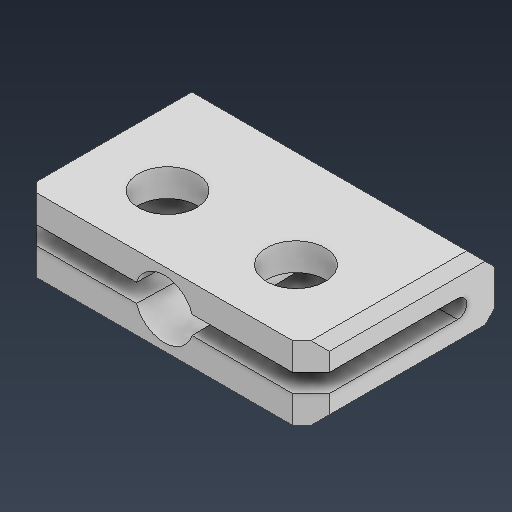
# Autodesk Inventor part: Sup_haste_corpo
Saved by Autodesk Inventor 2026.1 (Build 301233020, 233B)
## iProperties
Created: 2026-03-23
Part Number: Sup_haste_corpo
Material: Genérico
Document SubType Name: Modeling
Designer: celio
Density: 1 g/cm^3
Appearance: Padrão
Author: celio
Autodesk Inventor part; units mm, degrees
ref_plane "YZ Plane" through (0, 0, 0) normal (1, 0, 0) x (0, 1, 0)
ref_plane "XZ Plane" through (0, 0, 0) normal (0, 1, 0) x (-1, 0, 0)
ref_plane "XY Plane" through (0, 0, 0) normal (0, 0, 1) x (1, 0, 0)
sketch "Esboço1" plane through (0, 0, 0) normal (0, 1, 0) x (-1, 0, 0)
  line L0 (-8, -5) -> (8, -5)
  line L1 (8, -5) -> (8, 5)
  line L2 (8, 5) -> (-8, 5)
  line L3 (-8, 5) -> (-8, -5)
  line L4 (-8, -5) -> (8, 5) construction
  line L5 (8, -5) -> (-8, 5) construction
  point P0 (0, 0)
  dimension "d0" = 16
  dimension "d1" = 10
  constraints: 12 end point, 2 midpoint, 2 parallel, 1 horizontal, 1 perpendicular
  measures "d0" distance of L2.end L1.end
  measures "d1" distance of L1.end L0.end
extrude "Extrusão1" add sketch "Esboço1" along normal blind 4
sketch "Esboço2" plane through (8, 0, 5) normal (1, 0, 0) x (0, 0, -1)
  line L0 (0, 0) -> (0, 4) projected
  line L1 (10, 0) -> (10, 4) projected
  line L2 (-0.795, 1.5) -> (-0.795, 2.5)
  line L3 (-0.795, 2.5) -> (6.8544, 2.5)
  line L4 (6.8544, 1.5) -> (-0.795, 1.5)
  line L5 (-0.795, 2.5) -> (8, 2.5)
  line L6 (8.5, 2) -> (8.5, 2)
  line L7 (8, 1.5) -> (-0.795, 1.5)
  line L8 (-0.795, 1.5) -> (-0.795, 2.5)
  arc A0 (8.5, 2) -> (8, 2.5) centre (8, 2) ccw
  arc A1 (8, 1.5) -> (8.5, 2) centre (8, 2) ccw
  point P0 (5, 0)
  point P1 (0, 2.5)
  point P2 (0, 1.5)
  point P3 (8.5, 1.5)
  point P4 (8.5, 2.5)
  dimension "d8" = 1
  dimension "d26" = 9.295
  dimension "d27" = 1
  dimension "d28" = 0.5
  constraints: 14 end point, 4 point on circle, 4 point on line, 4 tangent, 3 parallel, 2 centre point, 2 horizontal, 2 perpendicular, 1 concentric
  measures "d8" distance of L2.start L2.end
  measures "d26" distance of point (8.5, 1.5) L7.end
  measures "d27" distance of point (8.5, 2.5) point (8.5, 1.5)
  measures "d28" radius of A0
chamfer "Chanfro1" distance 1 angle 45 2 edges at (-8, 2, 5) (8, 2, 5)
chamfer "Chanfro2" distance 1 angle 45 2 edges at (0, 4, -5) (0, 0, -5)
chamfer "Chanfro3" distance 0.5 angle 45 4 edges at (8, 4, 0) (8, 0, 0) (-8, 4, 0) (-8, 0, 0)
sketch "Esboço3" plane through (0, 4, 0) normal (0, 1, 0) x (1, 0, 0)
  line L0 (-7.5, -4.5) -> (-7.5, 4) projected
  line L1 (7, -5) -> (8, -4) projected
  line L2 (-7.5, 4) -> (7.5, 4)
  line L3 (7.5, 4) -> (7.5, -4.5)
  line L4 (7.5, -4.5) -> (-7.5, -4.5)
  line L5 (-7.5, -4.5) -> (-7.5, 4)
  line L6 (8, 1.8544) -> (-8, 1.8544) projected
  line L7 (-7.5, 1.8544) -> (7.5, 1.8544)
  line L8 (7.5, 1.8544) -> (7.5, -4.5)
  line L9 (7.5, -4.5) -> (-7.5, -4.5)
  line L10 (-7.5, -4.5) -> (-7.5, 1.8544)
  line L11 (-7.5, -1.3228) -> (7.5, -1.3228)
  line L12 (-7.5, -1.3228) -> (-3.5, -1.3228)
  circle A0 centre (-3.5, -1.3228) radius 1.6
  line L13 (7.5, -1.3228) -> (3.5, -1.3228)
  circle A1 centre (3.5, -1.3228) radius 1.6
  point P0 (0, 0)
  dimension "d20" = 4
  dimension "d21" = 3.2
  dimension "d22" = 4
  dimension "d23" = 3.2
  constraints: 22 end point, 4 parallel, 4 point on line, 3 midpoint, 2 centre point, 2 coincident, 2 horizontal, 2 perpendicular
  measures "d20" distance of L11.start L12.end
  measures "d21" diameter of A0
  measures "d22" distance of L11.end L13.end
  measures "d23" diameter of A1
extrude "Extrusão3" cut sketch "Esboço3" against normal through all contours A0 L11 | L11 A0 | A1 L11 | L11 A1
extrude "Extrusão4" cut sketch "Esboço2" against normal through all contours L0 L3 L5 A0 A1 L7 L4
sketch "Esboço4" plane through (8, 1, -5) normal (0, 0, -1) x (-1, 0, 0)
  line L0 (0, 1.5) -> (0, 2.5) projected
  line L1 (16, 0) -> (16, 2) projected
  line L2 (16, 2) -> (16, 0)
  line L3 (0, 0) -> (0, 2)
  circle A0 centre (8, 1) radius 1.35
  point P0 (8, -1)
  dimension "d31" = 2.7
  constraints: 4 end point, 1 centre point, 1 midpoint, 1 parallel
  measures "d31" diameter of A0
sketch "Esboço5" plane through (-7, 0, 5) normal (0, 0, 1) x (1, 0, 0)
  line L0 (0, 4) -> (-0.5, 4) projected
  line L1 (0, 0) -> (14, 0) projected
  line L2 (0, 4) -> (14, 4)
  line L3 (14, 4) -> (14, 0)
  line L4 (14, 0) -> (0, 0)
  line L5 (0, 0) -> (0, 4)
  circle A0 centre (7, 2) radius 1.6
  point P0 (7, 0)
  dimension "d32" = 3.2
  constraints: 8 end point, 2 parallel, 1 centre point, 1 horizontal, 1 perpendicular
  measures "d32" diameter of A0
loft "Transição1" cut profiles "Esboço4", "Esboço5" contours all / A0
